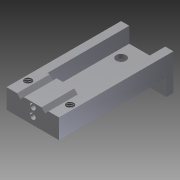
# Autodesk Inventor part: lickport_Holder_small
Saved by Autodesk Inventor 2012 SP2 (Build 160219200, 219)
## iProperties
Created: 2017-08-14
Part Number: lickport_Holder_small
Material: Default
Document SubType Name: Modeling
Designer: zhaox11
Density: 1 g/cm^3
Author: zhaox11
Autodesk Inventor part; units mm, degrees
ref_plane "YZ Plane" through (0, 0, 0) normal (1, 0, 0) x (0, 1, 0)
ref_plane "XZ Plane" through (0, 0, 0) normal (0, 1, 0) x (-1, 0, 0)
ref_plane "XY Plane" through (0, 0, 0) normal (0, 0, 1) x (1, 0, 0)
sketch "Sketch1" plane through (0, 0, 0) normal (0, 0, 1) x (1, 0, 0)
  line L0 (-10.16, 3.81) -> (10.16, 3.81)
  line L1 (10.16, 3.81) -> (10.16, -3.81)
  line L2 (10.16, -3.81) -> (-10.16, -3.81)
  line L3 (-10.16, -3.81) -> (-10.16, 3.81)
  point P0 (0, 0)
  dimension "d0" = 20.32
  dimension "d1" = 7.62
  dimension "d2" = 3.81
  dimension "d3" = 10.16
  constraints: 8 end point, 2 parallel, 1 horizontal, 1 perpendicular
  measures "d0" distance of L0.start L0.end
  measures "d1" distance of L0.end L1.end
  measures "d2" distance from line of point (0, 0) L0
  measures "d3" distance from line of point (0, 0) L1
extrude "Extrusion1" add sketch "Sketch1" against normal blind 12.7
sketch "Sketch2" plane through (0, 0, 0) normal (0, 0, 1) x (1, 0, 0)
  line L0 (-10.16, 3.81) -> (10.16, 3.81) projected
  circle A0 centre (0, 2.286) radius 1.143
  circle A1 centre (0, -0.889) radius 1.143
  circle A2 centre (-4.7625, 3.81) radius 0.9525
  circle A3 centre (4.7625, 3.81) radius 0.9525
  line L1 (-6.1095, 3.81) -> (-3.5541, 1.2546)
  line L2 (-3.4155, 3.81) -> (-5.4913, 1.7342)
  line L3 (3.4155, 3.81) -> (5.9385, 1.2869)
  line L4 (4.5051, 2.2056) -> (6.1095, 3.81)
  point P0 (0, 0)
  point P1 (-4.7625, 2.463)
  point P2 (4.7625, 2.463)
  dimension "d6" = 2.286
  dimension "d7" = 2.286
  dimension "d8" = 1.524
  dimension "d9" = 3.175
  dimension "d10" = 1.905
  dimension "d11" = 1.905
  dimension "d12" = 0
  dimension "d13" = 0
  dimension "d14" = 9.525
  dimension "d15" = 4.7625
  dimension "d16" = 45
  dimension "d17" = 45
  dimension "d18" = 45
  dimension "d19" = 45
  constraints: 8 end point, 8 point on line, 4 centre point, 4 tangent, 1 perpendicular
  measures "d6" diameter of A0
  measures "d7" diameter of A1
  measures "d8" distance from line of L0 A0.centre
  measures "d9" distance of A1.centre A0.centre
  measures "d10" diameter of A2
  measures "d11" diameter of A3
  measures "d12" distance from line of L0 A2.centre
  measures "d13" distance from line of L0 A3.centre
  measures "d14" distance of A3.centre A2.centre
  measures "d15" horizontal distance of point (0, 0) A2.centre
  measures "d16" angle of L0 L1
  measures "d17" angle of L0 L2
  measures "d18" angle of L0 L4
  measures "d19" angle of L0 L3
extrude "Extrusion3" cut sketch "Sketch2" against normal blind 12.7 contours L0 A3 L3 | A2 L0 | L0 L2 A2 | A2 L1 L0 | L2 L1 A2 | L0 A3 | A3 L4 L3 | L0 L4 A3 | A0 | A1 picked at (-4.7051, 3.27) picked at (4.6576, 3.5103)
sketch "Sketch3" plane through (-10.16, 3.81, 0) normal (0, 1, 0) x (1, 0, 0)
  line L0 (4.0505, 12.7) -> (0, 12.7) projected
  line L1 (0, 0) -> (0, 12.7) projected
  line L2 (0, 0) -> (4.0505, 0) projected
  circle A0 centre (2.0252, 6.35) radius 1.4224
  point P0 (10.16, 0)
  dimension "d24" = 2.8448
  dimension "d25" = 6.35
  dimension "d26" = 12.7
  dimension "d31" = 4.0505
  dimension "d32" = 2.0252
  constraints: 1 centre point
  measures "d24" diameter of A0
  measures "d25" distance from line of L2 A0.centre
  measures "d26" distance between parallel lines of L2 L0
  measures "d31" distance of L0.start L0.end
  measures "d32" distance from line of A0.centre L1
sketch "Sketch4" plane through (10.16, 3.81, 0) normal (0, 1, 0) x (1, 0, 0)
  line L0 (-4.0505, 0) -> (0, 0) projected
  line L1 (0, 0) -> (0, 12.7) projected
  circle A0 centre (-2.0252, 6.35) radius 1.4224
  point P0 (-4.0505, 12.7)
  point P1 (-10.16, 0)
  dimension "d27" = 2.8448
  dimension "d28" = 6.35
  dimension "d29" = 4.0505
  dimension "d30" = 2.0252
  constraints: 1 centre point
  measures "d27" diameter of A0
  measures "d28" distance from line of L0 A0.centre
  measures "d29" distance of L1.end point (-4.05, 12.7)
  measures "d30" distance from line of L1 A0.centre
extrude "Extrusion4" cut sketch "Sketch3" against normal blind 12.7
extrude "Extrusion5" cut sketch "Sketch4" against normal blind 12.7
sketch "Sketch5" plane through (0, 0, -12.7) normal (0, 0, -1) x (-1, 0, 0)
  line L0 (-10.16, -3.81) -> (-10.16, 3.81) projected
  line L1 (10.16, -3.81) -> (-10.16, -3.81) projected
  line L2 (10.16, 3.81) -> (10.16, -3.81) projected
  line L3 (-10.16, 3.81) -> (-6.985, 3.81)
  line L4 (-6.985, 3.81) -> (-6.985, -3.81)
  line L5 (-6.985, -3.81) -> (-10.16, -3.81)
  line L6 (-10.16, -3.81) -> (-10.16, 3.81)
  line L7 (10.16, 3.81) -> (6.985, 3.81)
  line L8 (6.985, 3.81) -> (6.985, -3.81)
  line L9 (6.985, -3.81) -> (10.16, -3.81)
  line L10 (10.16, -3.81) -> (10.16, 3.81)
  line L11 (-10.16, -2.2225) -> (6.985, -2.2225)
  line L12 (6.985, -2.2225) -> (6.985, -3.81)
  line L13 (6.985, -3.81) -> (-10.16, -3.81)
  line L14 (-10.16, -3.81) -> (-10.16, -2.2225)
  point P0 (0, 0)
  dimension "d37" = 3.175
  dimension "d38" = 3.175
  dimension "d39" = 1.5875
  constraints: 24 end point, 6 parallel, 3 horizontal, 3 perpendicular, 3 point on line
  measures "d37" distance between parallel lines of L4 L0
  measures "d38" distance between parallel lines of L2 L8
  measures "d39" distance between parallel lines of L13 L11
extrude "Extrusion6" add sketch "Sketch5" along normal blind 31.75
thread "Thread1" size "4-40 UNC" class "2B" standard "ANSI Unified Screw Threads" full length
thread "Thread2" size "4-40 UNC" class "2B" standard "ANSI Unified Screw Threads" full length
sketch "Sketch8" plane through (-10.16, -3.81, 0) normal (0, -1, 0) x (1, 0, 0)
  line L0 (20.32, 0) -> (20.32, -44.45) projected
  line L1 (0, -44.45) -> (20.32, -44.45)
  line L2 (20.32, -44.45) -> (20.32, -41.656)
  line L3 (20.32, -41.656) -> (0, -41.656)
  line L4 (0, -41.656) -> (0, -44.45)
  point P0 (10.16, 0)
  dimension "d58" = 2.794
  constraints: 8 end point, 2 parallel, 1 horizontal, 1 perpendicular, 1 point on line
  measures "d58" distance between parallel lines of L1 L3
extrude "Extrusion9" add sketch "Sketch8" along normal blind 6.35
sketch "Sketch9" plane through (-10.16, -3.81, -41.656) normal (0, 0, 1) x (1, 0, 0)
  line L0 (0, 0) -> (20.32, 0) projected
  line L1 (0, 0) -> (0, -6.35) projected
  circle A0 centre (10.16, -3.175) radius 1.524
  point P0 (20.32, -6.35)
  point P1 (10.16, 3.81)
  dimension "d61" = 3.048
  dimension "d62" = 20.32
  dimension "d63" = 6.35
  dimension "d64" = 3.175
  dimension "d65" = 10.16
  constraints: 1 centre point
  measures "d61" diameter of A0
  measures "d62" distance of L1.end point (20.32, -6.35)
  measures "d63" distance of L0.start L1.end
  measures "d64" distance from line of L0 A0.centre
  measures "d65" distance from line of L1 A0.centre
extrude "Extrusion10" cut sketch "Sketch9" against normal blind 7.62
sketch "Sketch10" plane through (-6.985, -2.2225, -12.7) normal (0, 1, 0) x (1, 0, 0)
  line L0 (13.97, 0) -> (13.97, 31.75) projected
  line L1 (0, 0) -> (0, 31.75) projected
  line L2 (13.97, 0) -> (0, 0) projected
  circle A0 centre (3.175, 25.4) radius 1.905
  circle A1 centre (10.795, 25.4) radius 1.905
  point P0 (6.985, -12.7)
  dimension "d68" = 3.81
  dimension "d69" = 3.81
  dimension "d70" = 3.175
  dimension "d71" = 3.175
  dimension "d72" = 25.4
  dimension "d73" = 25.4
  constraints: 2 centre point
  measures "d68" diameter of A0
  measures "d69" diameter of A1
  measures "d70" distance from line of L1 A0.centre
  measures "d71" distance from line of L0 A1.centre
  measures "d72" distance from line of L2 A0.centre
  measures "d73" distance from line of L2 A1.centre
extrude "Extrusion11" cut sketch "Sketch10" against normal blind 7.62
equation "\"d2\" = 0.5 * d1"
equation "\"d3\" = 0.5 * d0"
equation "\"d7\" = d6"
equation "\"d15\" = 0.5 * d14"
equation "\"d25\" = 0.5 * d26"
equation "\"d32\" = 0.5 * d31"
equation "\"d28\" = d25"
equation "\"d30\" = 0.5 * d29"
equation "\"d38\" = d37"
equation "\"d64\" = 0.5 * d63"
equation "\"d65\" = 0.5 * d62"
equation "\"d73\" = d72"
body "Solid1"
